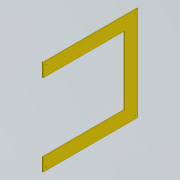
# Autodesk Inventor part: FrameCentre
Saved by Autodesk Inventor 2016 (Build 200138000, 138)
## iProperties
Created: 2016-08-20
Part Number: FrameCentre
Material: Dibond Yellow
Document SubType Name: Modeling
Designer: Sam
Density: 1 g/cm^3
Appearance: Generic(1)
Author: Sam
Autodesk Inventor part; units mm, degrees
ref_plane "YZ Plane" through (0, 0, 0) normal (1, 0, 0) x (0, 1, 0)
ref_plane "XZ Plane" through (0, 0, 0) normal (0, 1, 0) x (-1, 0, 0)
ref_plane "XY Plane" through (0, 0, 0) normal (0, 0, 1) x (1, 0, 0)
sketch "Sketch1" plane through (0, 0, 0) normal (1, 0, 0) x (0, 1, 0)
  line L0 (0, 0) -> (360, 0)
  line L1 (360, 0) -> (360, -360)
  line L2 (360, -360) -> (0, -360)
  line L3 (0, -360) -> (0, -310)
  line L4 (0, -50) -> (310, -50)
  line L5 (310, -50) -> (310, -310)
  line L6 (310, -310) -> (0, -310)
  line L7 (0, -310) -> (0, -50)
  line L8 (0, -50) -> (0, 0)
  line L9 (0, -310) -> (0, -50)
  dimension "d4" = 360
  dimension "d5" = 360
  dimension "d6" = 310
  dimension "d7" = 260
  constraints: 20 end point, 6 parallel, 2 horizontal, 2 perpendicular
  measures "d4" distance of L1.end L2.end
  measures "d5" distance of L0.end L1.end
  measures "d6" distance of L5.end L3.end
  measures "d7" distance of L4.end L5.end
extrude "Extrusion1" add sketch "Sketch1" along normal blind 3 contours L0 L1 L2 L3 L6 L5 L4 L8
hole "Hole1" at (3, 348, -12) direction (-1, 0, 0) diameter 4 end through all
hole "Hole2" at (3, 348, -348) direction (-1, 0, 0) diameter 4 end through all
hole "Hole3" at (3, 12, -348) direction (-1, 0, 0) diameter 4 end through all
hole "Hole4" at (3, 12, -12) direction (-1, 0, 0) diameter 4 end through all
body "Solid1"
